Autodesk Inventor part; units mm, degrees
(part 2 of 4)
  spline S285 degree 2 poles (64.2281, 27.9943) (64.3898, 27.9943) (64.7103, 28.0368) (64.8067, 28.0822) knots 0 0 0 1 2 2 2
  spline S286 degree 2 poles (64.8067, 28.0822) (64.9173, 28.1389) (65.0421, 28.329) (65.0534, 28.4708) knots 0 0 0 1 2 2 2
  line L243 (65.0534, 28.4708) -> (65.8192, 28.4708)
  line L244 (65.8192, 28.4708) -> (65.8192, 25.5721)
  line L245 (65.8192, 25.5721) -> (66.5397, 25.5721)
  line L246 (66.5397, 25.5721) -> (66.5397, 24.9623)
  line L247 (69.1803, 28.6183) -> (67.7876, 24.2021)
  line L248 (67.7876, 24.2021) -> (67.1126, 24.2021)
  line L249 (67.1126, 24.2021) -> (68.5024, 28.6183)
  line L250 (68.5024, 28.6183) -> (69.1803, 28.6183)
  spline S287 degree 2 poles (71.4833, 24.8942) (70.6949, 24.8942) (69.7702, 25.8472) (69.7702, 26.7094) knots 0 0 0 1 2 2 2
  spline S288 degree 2 poles (69.7702, 26.7094) (69.7702, 27.5405) (70.6977, 28.5303) (71.4862, 28.5303) knots 0 0 0 1 2 2 2
  spline S289 degree 2 poles (71.4862, 28.5303) (71.6932, 28.5303) (72.0279, 28.4821) (72.1811, 28.4424) knots 0 0 0 1 2 2 2
  spline S290 degree 2 poles (72.1811, 28.4424) (72.3002, 28.4055) (72.581, 28.2836) (72.6689, 28.2382) knots 0 0 0 1 2 2 2
  line L251 (72.6689, 28.2382) -> (72.6689, 27.4043)
  line L252 (72.6689, 27.4043) -> (72.581, 27.4043)
  spline S291 degree 2 poles (72.581, 27.4043) (72.5158, 27.461) (72.3229, 27.6199) (72.2009, 27.6936) knots 0 0 0 1 2 2 2
  spline S292 degree 2 poles (72.2009, 27.6936) (72.079, 27.7702) (71.7868, 27.8751) (71.6252, 27.8751) knots 0 0 0 1 2 2 2
  spline S293 degree 2 poles (71.6252, 27.8751) (71.4351, 27.8751) (71.1203, 27.756) (70.9757, 27.6057) knots 0 0 0 1 2 2 2
  spline S294 degree 2 poles (70.9757, 27.6057) (70.8452, 27.4724) (70.6778, 27.0157) (70.6778, 26.7066) knots 0 0 0 1 2 2 2
  spline S295 degree 2 poles (70.6778, 26.7066) (70.6778, 26.3804) (70.8509, 25.9351) (70.9927, 25.799) knots 0 0 0 1 2 2 2
  spline S296 degree 2 poles (70.9927, 25.799) (71.1288, 25.6657) (71.4635, 25.5494) (71.6308, 25.5494) knots 0 0 0 1 2 2 2
  spline S297 degree 2 poles (71.6308, 25.5494) (71.8039, 25.5494) (72.1187, 25.6657) (72.2265, 25.7366) knots 0 0 0 1 2 2 2
  spline S298 degree 2 poles (72.2265, 25.7366) (72.3456, 25.8075) (72.5243, 25.9578) (72.5895, 26.0174) knots 0 0 0 1 2 2 2
  line L253 (72.5895, 26.0174) -> (72.6689, 26.0174)
  line L254 (72.6689, 26.0174) -> (72.6689, 25.1948)
  spline S299 degree 2 poles (72.6689, 25.1948) (72.5725, 25.1495) (72.3201, 25.036) (72.1839, 24.9963) knots 0 0 0 1 2 2 2
  spline S300 degree 2 poles (72.1839, 24.9963) (72.0194, 24.9452) (71.7329, 24.8942) (71.4833, 24.8942) knots 0 0 0 1 2 2 2
  spline S301 degree 2 poles (74.5948, 25.2431) (74.5097, 25.1721) (74.3764, 25.0587) (74.2629, 25.002) knots 0 0 0 1 2 2 2
  spline S302 degree 2 poles (74.2629, 25.002) (74.1523, 24.9481) (73.9424, 24.8914) (73.7552, 24.8914) knots 0 0 0 1 2 2 2
  spline S303 degree 2 poles (73.7552, 24.8914) (73.4035, 24.8914) (72.9412, 25.3622) (72.9412, 25.7196) knots 0 0 0 1 2 2 2
  spline S304 degree 2 poles (72.9412, 25.7196) (72.9412, 26.0117) (73.1766, 26.3747) (73.3979, 26.4797) knots 0 0 0 1 2 2 2
  spline S305 degree 2 poles (73.3979, 26.4797) (73.6219, 26.5875) (74.2431, 26.6726) (74.6004, 26.6952) knots 0 0 0 1 2 2 2
  line L255 (74.6004, 26.6952) -> (74.6004, 26.7094)
  spline S306 degree 2 poles (74.6004, 26.7094) (74.6004, 26.9278) (74.2771, 27.0952) (73.9538, 27.0952) knots 0 0 0 1 2 2 2
  spline S307 degree 2 poles (73.9538, 27.0952) (73.8091, 27.0952) (73.4177, 26.9902) (73.2333, 26.908) knots 0 0 0 1 2 2 2
  line L256 (73.2333, 26.908) -> (73.1624, 26.908)
  line L257 (73.1624, 26.908) -> (73.1624, 27.5461)
  spline S308 degree 2 poles (73.1624, 27.5461) (73.2844, 27.5802) (73.829, 27.6766) (74.1069, 27.6766) knots 0 0 0 1 2 2 2
  spline S309 degree 2 poles (74.1069, 27.6766) (74.7876, 27.6766) (75.4116, 27.2228) (75.4116, 26.7576) knots 0 0 0 1 2 2 2
  line L258 (75.4116, 26.7576) -> (75.4116, 24.9623)
  line L259 (75.4116, 24.9623) -> (74.5948, 24.9623)
  line L260 (74.5948, 24.9623) -> (74.5948, 25.2431)
  line L261 (74.5948, 25.6515) -> (74.5948, 26.1989)
  spline S310 degree 2 poles (74.5948, 26.1989) (74.3849, 26.179) (74.1268, 26.1478) (74.002, 26.1025) knots 0 0 0 1 2 2 2
  spline S311 degree 2 poles (74.002, 26.1025) (73.8914, 26.0656) (73.7722, 25.9124) (73.7722, 25.7876) knots 0 0 0 1 2 2 2
  spline S312 degree 2 poles (73.7722, 25.7876) (73.7722, 25.6033) (73.9736, 25.4643) (74.1693, 25.4643) knots 0 0 0 1 2 2 2
  spline S313 degree 2 poles (74.1693, 25.4643) (74.2771, 25.4643) (74.504, 25.5636) (74.5948, 25.6515) knots 0 0 0 1 2 2 2
  line L262 (76.844, 24.9623) -> (76.0214, 24.9623)
  line L263 (76.0214, 24.9623) -> (76.0214, 28.6183)
  line L264 (76.0214, 28.6183) -> (76.844, 28.6183)
  line L265 (76.844, 28.6183) -> (76.844, 24.9623)
  spline S314 degree 2 poles (80.0064, 26.2811) (80.0064, 25.6288) (79.2945, 24.88) (78.645, 24.88) knots 0 0 0 1 2 2 2
  spline S315 degree 2 poles (78.645, 24.88) (77.9983, 24.88) (77.2808, 25.6288) (77.2808, 26.2811) knots 0 0 0 1 2 2 2
  spline S316 degree 2 poles (77.2808, 26.2811) (77.2808, 26.9392) (77.9983, 27.6851) (78.645, 27.6851) knots 0 0 0 1 2 2 2
  spline S317 degree 2 poles (78.645, 27.6851) (79.2917, 27.6851) (80.0064, 26.9363) (80.0064, 26.2811) knots 0 0 0 1 2 2 2
  spline S318 degree 2 poles (79.1641, 26.2755) (79.1641, 26.5109) (79.0875, 26.8257) (79.0194, 26.9193) knots 0 0 0 1 2 2 2
  spline S319 degree 2 poles (79.0194, 26.9193) (78.9457, 27.0186) (78.7613, 27.0952) (78.645, 27.0952) knots 0 0 0 1 2 2 2
  spline S320 degree 2 poles (78.645, 27.0952) (78.5316, 27.0952) (78.3529, 27.0271) (78.2791, 26.9307) knots 0 0 0 1 2 2 2
  spline S321 degree 2 poles (78.2791, 26.9307) (78.2082, 26.8399) (78.1231, 26.5194) (78.1231, 26.2755) knots 0 0 0 1 2 2 2
  spline S322 degree 2 poles (78.1231, 26.2755) (78.1231, 26.0344) (78.2026, 25.7366) (78.2678, 25.6458) knots 0 0 0 1 2 2 2
  spline S323 degree 2 poles (78.2678, 25.6458) (78.333, 25.555) (78.5316, 25.47) (78.6507, 25.47) knots 0 0 0 1 2 2 2
  spline S324 degree 2 poles (78.6507, 25.47) (78.75, 25.47) (78.9542, 25.555) (79.0166, 25.6401) knots 0 0 0 1 2 2 2
  spline S325 degree 2 poles (79.0166, 25.6401) (79.0875, 25.7394) (79.1641, 26.0259) (79.1641, 26.2755) knots 0 0 0 1 2 2 2
  line L266 (82.2159, 26.8229) -> (82.1479, 26.8229)
  spline S326 degree 2 poles (82.1479, 26.8229) (82.0996, 26.8399) (81.921, 26.8569) (81.8132, 26.8569) knots 0 0 0 1 2 2 2
  spline S327 degree 2 poles (81.8132, 26.8569) (81.6855, 26.8569) (81.3991, 26.7803) (81.2658, 26.7293) knots 0 0 0 1 2 2 2
  line L267 (81.2658, 26.7293) -> (81.2658, 24.9623)
  line L268 (81.2658, 24.9623) -> (80.4432, 24.9623)
  line L269 (80.4432, 24.9623) -> (80.4432, 27.6029)
  line L270 (80.4432, 27.6029) -> (81.2658, 27.6029)
  line L271 (81.2658, 27.6029) -> (81.2658, 27.2228)
  spline S328 degree 2 poles (81.2658, 27.2228) (81.3225, 27.2739) (81.521, 27.4327) (81.6033, 27.4809) knots 0 0 0 1 2 2 2
  spline S329 degree 2 poles (81.6033, 27.4809) (81.694, 27.5348) (81.9323, 27.6114) (82.0372, 27.6114) knots 0 0 0 1 2 2 2
  spline S330 degree 2 poles (82.0372, 27.6114) (82.0769, 27.6114) (82.1762, 27.6057) (82.2159, 27.6029) knots 0 0 0 1 2 2 2
  line L272 (82.2159, 27.6029) -> (82.2159, 26.8229)
  line L273 (83.3533, 24.9623) -> (82.5308, 24.9623)
  line L274 (82.5308, 24.9623) -> (82.5308, 27.6029)
  line L275 (82.5308, 27.6029) -> (83.3533, 27.6029)
  line L276 (83.3533, 27.6029) -> (83.3533, 24.9623)
  line L277 (83.3788, 27.9801) -> (82.5081, 27.9801)
  line L278 (82.5081, 27.9801) -> (82.5081, 28.6211)
  line L279 (82.5081, 28.6211) -> (83.3788, 28.6211)
  line L280 (83.3788, 28.6211) -> (83.3788, 27.9801)
  line L281 (87.1341, 24.9623) -> (87.1341, 26.2811)
  spline S331 degree 2 poles (87.1341, 26.2811) (87.1341, 26.4768) (87.1199, 26.7435) (87.0859, 26.8286) knots 0 0 0 1 2 2 2
  spline S332 degree 2 poles (87.0859, 26.8286) (87.049, 26.9136) (86.9015, 26.9902) (86.7682, 26.9902) knots 0 0 0 1 2 2 2
  spline S333 degree 2 poles (86.7682, 26.9902) (86.6746, 26.9902) (86.4931, 26.908) (86.3853, 26.8314) knots 0 0 0 1 2 2 2
  line L282 (86.3853, 26.8314) -> (86.3853, 24.9623)
  line L283 (86.3853, 24.9623) -> (85.5571, 24.9623)
  line L284 (85.5571, 24.9623) -> (85.5571, 26.2811)
  spline S334 degree 2 poles (85.5571, 26.2811) (85.5571, 26.474) (85.5401, 26.7435) (85.506, 26.8286) knots 0 0 0 1 2 2 2
  spline S335 degree 2 poles (85.506, 26.8286) (85.4692, 26.9136) (85.3217, 26.9902) (85.1884, 26.9902) knots 0 0 0 1 2 2 2
  spline S336 degree 2 poles (85.1884, 26.9902) (85.0891, 26.9902) (84.8934, 26.8966) (84.8026, 26.8314) knots 0 0 0 1 2 2 2
  line L285 (84.8026, 26.8314) -> (84.8026, 24.9623)
  line L286 (84.8026, 24.9623) -> (83.9801, 24.9623)
  line L287 (83.9801, 24.9623) -> (83.9801, 27.6029)
  line L288 (83.9801, 27.6029) -> (84.8026, 27.6029)
  line L289 (84.8026, 27.6029) -> (84.8026, 27.3107)
  spline S337 degree 2 poles (84.8026, 27.3107) (85.004, 27.4809) (85.3642, 27.6738) (85.5883, 27.6738) knots 0 0 0 1 2 2 2
  spline S338 degree 2 poles (85.5883, 27.6738) (85.8294, 27.6738) (86.1981, 27.444) (86.2945, 27.2143) knots 0 0 0 1 2 2 2
  spline S339 degree 2 poles (86.2945, 27.2143) (86.5299, 27.4355) (86.9497, 27.6738) (87.1653, 27.6738) knots 0 0 0 1 2 2 2
  spline S340 degree 2 poles (87.1653, 27.6738) (87.3496, 27.6738) (87.6418, 27.5575) (87.741, 27.4384) knots 0 0 0 1 2 2 2
  spline S341 degree 2 poles (87.741, 27.4384) (87.8517, 27.3107) (87.9623, 26.9619) (87.9623, 26.6811) knots 0 0 0 1 2 2 2
  line L290 (87.9623, 26.6811) -> (87.9623, 24.9623)
  line L291 (87.9623, 24.9623) -> (87.1341, 24.9623)
  spline S342 degree 2 poles (89.925, 24.8914) (89.1762, 24.8914) (88.3792, 25.6061) (88.3792, 26.267) knots 0 0 0 1 2 2 2
  spline S343 degree 2 poles (88.3792, 26.267) (88.3792, 26.9136) (89.1223, 27.6851) (89.7917, 27.6851) knots 0 0 0 1 2 2 2
  spline S344 degree 2 poles (89.7917, 27.6851) (90.3958, 27.6851) (91.0085, 27.0299) (91.0085, 26.423) knots 0 0 0 1 2 2 2
  line L292 (91.0085, 26.423) -> (91.0085, 26.1251)
  line L293 (91.0085, 26.1251) -> (89.2017, 26.1251)
  spline S345 degree 2 poles (89.2017, 26.1251) (89.2131, 25.9408) (89.3464, 25.6969) (89.4542, 25.6231) knots 0 0 0 1 2 2 2
  spline S346 degree 2 poles (89.4542, 25.6231) (89.5591, 25.5494) (89.8427, 25.487) (90.0101, 25.487) knots 0 0 0 1 2 2 2
  spline S347 degree 2 poles (90.0101, 25.487) (90.1519, 25.487) (90.4299, 25.5494) (90.5462, 25.6033) knots 0 0 0 1 2 2 2
  spline S348 degree 2 poles (90.5462, 25.6033) (90.6483, 25.6458) (90.8184, 25.7508) (90.8723, 25.7905) knots 0 0 0 1 2 2 2
  line L294 (90.8723, 25.7905) -> (90.9603, 25.7905)
  line L295 (90.9603, 25.7905) -> (90.9603, 25.1097)
  spline S349 degree 2 poles (90.9603, 25.1097) (90.8581, 25.07) (90.6936, 25.002) (90.5462, 24.9679) knots 0 0 0 1 2 2 2
  spline S350 degree 2 poles (90.5462, 24.9679) (90.4128, 24.9311) (90.1292, 24.8914) (89.925, 24.8914) knots 0 0 0 1 2 2 2
  spline S351 degree 2 poles (90.1973, 26.6215) (90.1916, 26.8824) (89.9619, 27.1576) (89.7265, 27.1576) knots 0 0 0 1 2 2 2
  spline S352 degree 2 poles (89.7265, 27.1576) (89.4854, 27.1576) (89.2131, 26.8683) (89.1989, 26.6215) knots 0 0 0 1 2 2 2
  line L296 (89.1989, 26.6215) -> (90.1973, 26.6215)
  spline S353 degree 2 poles (92.4408, 24.9112) (91.9388, 24.9112) (91.4793, 25.3253) (91.4793, 25.7961) knots 0 0 0 1 2 2 2
  line L297 (91.4793, 25.7961) -> (91.4793, 27.0299)
  line L298 (91.4793, 27.0299) -> (91.1645, 27.0299)
  line L299 (91.1645, 27.0299) -> (91.1645, 27.6029)
  line L300 (91.1645, 27.6029) -> (91.4793, 27.6029)
  line L301 (91.4793, 27.6029) -> (91.4793, 28.3573)
  line L302 (91.4793, 28.3573) -> (92.3018, 28.3573)
  line L303 (92.3018, 28.3573) -> (92.3018, 27.6029)
  line L304 (92.3018, 27.6029) -> (93.096, 27.6029)
  line L305 (93.096, 27.6029) -> (93.096, 27.0299)
  line L306 (93.096, 27.0299) -> (92.3018, 27.0299)
  line L307 (92.3018, 27.0299) -> (92.3018, 26.0911)
  spline S354 degree 2 poles (92.3018, 26.0911) (92.3018, 25.9521) (92.3075, 25.7451) (92.3415, 25.6628) knots 0 0 0 1 2 2 2
  spline S355 degree 2 poles (92.3415, 25.6628) (92.3756, 25.5806) (92.5429, 25.4841) (92.7017, 25.4841) knots 0 0 0 1 2 2 2
  spline S356 degree 2 poles (92.7017, 25.4841) (92.7698, 25.4841) (92.9825, 25.5409) (93.0251, 25.5636) knots 0 0 0 1 2 2 2
  line L308 (93.0251, 25.5636) -> (93.096, 25.5636)
  line L309 (93.096, 25.5636) -> (93.096, 24.985)
  spline S357 degree 2 poles (93.096, 24.985) (92.9627, 24.9509) (92.662, 24.9112) (92.4408, 24.9112) knots 0 0 0 1 2 2 2
  line L310 (95.2034, 26.8229) -> (95.1353, 26.8229)
  spline S358 degree 2 poles (95.1353, 26.8229) (95.0871, 26.8399) (94.9084, 26.8569) (94.8006, 26.8569) knots 0 0 0 1 2 2 2
  spline S359 degree 2 poles (94.8006, 26.8569) (94.673, 26.8569) (94.3865, 26.7803) (94.2532, 26.7293) knots 0 0 0 1 2 2 2
  line L311 (94.2532, 26.7293) -> (94.2532, 24.9623)
  line L312 (94.2532, 24.9623) -> (93.4307, 24.9623)
  line L313 (93.4307, 24.9623) -> (93.4307, 27.6029)
  line L314 (93.4307, 27.6029) -> (94.2532, 27.6029)
  line L315 (94.2532, 27.6029) -> (94.2532, 27.2228)
  spline S360 degree 2 poles (94.2532, 27.2228) (94.3099, 27.2739) (94.5085, 27.4327) (94.5907, 27.4809) knots 0 0 0 1 2 2 2
  spline S361 degree 2 poles (94.5907, 27.4809) (94.6815, 27.5348) (94.9197, 27.6114) (95.0247, 27.6114) knots 0 0 0 1 2 2 2
  spline S362 degree 2 poles (95.0247, 27.6114) (95.0644, 27.6114) (95.1637, 27.6057) (95.2034, 27.6029) knots 0 0 0 1 2 2 2
  line L316 (95.2034, 27.6029) -> (95.2034, 26.8229)
  spline S363 degree 2 poles (98.051, 26.2811) (98.051, 25.6288) (97.3391, 24.88) (96.6896, 24.88) knots 0 0 0 1 2 2 2
  spline S364 degree 2 poles (96.6896, 24.88) (96.0429, 24.88) (95.3253, 25.6288) (95.3253, 26.2811) knots 0 0 0 1 2 2 2
  spline S365 degree 2 poles (95.3253, 26.2811) (95.3253, 26.9392) (96.0429, 27.6851) (96.6896, 27.6851) knots 0 0 0 1 2 2 2
  spline S366 degree 2 poles (96.6896, 27.6851) (97.3363, 27.6851) (98.051, 26.9363) (98.051, 26.2811) knots 0 0 0 1 2 2 2
  spline S367 degree 2 poles (97.2086, 26.2755) (97.2086, 26.5109) (97.1321, 26.8257) (97.064, 26.9193) knots 0 0 0 1 2 2 2
  spline S368 degree 2 poles (97.064, 26.9193) (96.9902, 27.0186) (96.8059, 27.0952) (96.6896, 27.0952) knots 0 0 0 1 2 2 2
  spline S369 degree 2 poles (96.6896, 27.0952) (96.5761, 27.0952) (96.3974, 27.0271) (96.3237, 26.9307) knots 0 0 0 1 2 2 2
  spline S370 degree 2 poles (96.3237, 26.9307) (96.2528, 26.8399) (96.1677, 26.5194) (96.1677, 26.2755) knots 0 0 0 1 2 2 2
  spline S371 degree 2 poles (96.1677, 26.2755) (96.1677, 26.0344) (96.2471, 25.7366) (96.3124, 25.6458) knots 0 0 0 1 2 2 2
  spline S372 degree 2 poles (96.3124, 25.6458) (96.3776, 25.555) (96.5761, 25.47) (96.6953, 25.47) knots 0 0 0 1 2 2 2
  spline S373 degree 2 poles (96.6953, 25.47) (96.7945, 25.47) (96.9987, 25.555) (97.0611, 25.6401) knots 0 0 0 1 2 2 2
  spline S374 degree 2 poles (97.0611, 25.6401) (97.1321, 25.7394) (97.2086, 26.0259) (97.2086, 26.2755) knots 0 0 0 1 2 2 2
  spline S375 degree 2 poles (27.7919, 16.1032) (27.5359, 15.9989) (26.7174, 15.7998) (26.3191, 15.7998) knots 0 0 0 1 2 2 2
  spline S376 degree 2 poles (26.3191, 15.7998) (25.3994, 15.7998) (24.3091, 16.8617) (24.3091, 17.8351) knots 0 0 0 1 2 2 2
  spline S377 degree 2 poles (24.3091, 17.8351) (24.3091, 18.7517) (25.3994, 19.8578) (26.3476, 19.8578) knots 0 0 0 1 2 2 2
  spline S378 degree 2 poles (26.3476, 19.8578) (26.8374, 19.8578) (27.4506, 19.6714) (27.7761, 19.5133) knots 0 0 0 1 2 2 2
  line L317 (27.7761, 19.5133) -> (27.7761, 18.5968)
  line L318 (27.7761, 18.5968) -> (27.6876, 18.5968)
  spline S379 degree 2 poles (27.6876, 18.5968) (27.6181, 18.6505) (27.3526, 18.856) (27.2262, 18.9255) knots 0 0 0 1 2 2 2
  spline S380 degree 2 poles (27.2262, 18.9255) (27.0808, 19.0108) (26.6952, 19.1309) (26.4803, 19.1309) knots 0 0 0 1 2 2 2
  spline S381 degree 2 poles (26.4803, 19.1309) (26.2306, 19.1309) (25.8166, 18.9729) (25.6554, 18.8117) knots 0 0 0 1 2 2 2
  spline S382 degree 2 poles (25.6554, 18.8117) (25.5006, 18.6537) (25.3204, 18.1701) (25.3204, 17.8509) knots 0 0 0 1 2 2 2
  spline S383 degree 2 poles (25.3204, 17.8509) (25.3204, 17.1683) (26.0062, 16.5172) (26.5973, 16.5172) knots 0 0 0 1 2 2 2
  spline S384 degree 2 poles (26.5973, 16.5172) (26.651, 16.5172) (26.79, 16.5235) (26.8438, 16.5267) knots 0 0 0 1 2 2 2
  line L319 (26.8438, 16.5267) -> (26.8438, 17.2947)
  line L320 (26.8438, 17.2947) -> (26.0884, 17.2947)
  line L321 (26.0884, 17.2947) -> (26.0884, 18.0248)
  line L322 (26.0884, 18.0248) -> (27.7919, 18.0248)
  line L323 (27.7919, 18.0248) -> (27.7919, 16.1032)
  spline S385 degree 2 poles (30.099, 16.1949) (30.0042, 16.1158) (29.8557, 15.9894) (29.7293, 15.9262) knots 0 0 0 1 2 2 2
  spline S386 degree 2 poles (29.7293, 15.9262) (29.606, 15.8662) (29.3721, 15.803) (29.1635, 15.803) knots 0 0 0 1 2 2 2
  spline S387 degree 2 poles (29.1635, 15.803) (28.7716, 15.803) (28.2565, 16.3276) (28.2565, 16.7258) knots 0 0 0 1 2 2 2
  spline S388 degree 2 poles (28.2565, 16.7258) (28.2565, 17.0513) (28.5188, 17.4559) (28.7653, 17.5728) knots 0 0 0 1 2 2 2
  spline S389 degree 2 poles (28.7653, 17.5728) (29.015, 17.6929) (29.7071, 17.7877) (30.1054, 17.813) knots 0 0 0 1 2 2 2
  line L324 (30.1054, 17.813) -> (30.1054, 17.8288)
  spline S390 degree 2 poles (30.1054, 17.8288) (30.1054, 18.0722) (29.7451, 18.2586) (29.3848, 18.2586) knots 0 0 0 1 2 2 2
  spline S391 degree 2 poles (29.3848, 18.2586) (29.2236, 18.2586) (28.7874, 18.1417) (28.582, 18.05) knots 0 0 0 1 2 2 2
  line L325 (28.582, 18.05) -> (28.503, 18.05)
  line L326 (28.503, 18.05) -> (28.503, 18.7611)
  spline S392 degree 2 poles (28.503, 18.7611) (28.6389, 18.7991) (29.2457, 18.9065) (29.5554, 18.9065) knots 0 0 0 1 2 2 2
  spline S393 degree 2 poles (29.5554, 18.9065) (30.3139, 18.9065) (31.0092, 18.4009) (31.0092, 17.8825) knots 0 0 0 1 2 2 2
  line L327 (31.0092, 17.8825) -> (31.0092, 15.882)
  line L328 (31.0092, 15.882) -> (30.099, 15.882)
  line L329 (30.099, 15.882) -> (30.099, 16.1949)
  line L330 (30.099, 16.65) -> (30.099, 17.2599)
  spline S394 degree 2 poles (30.099, 17.2599) (29.8652, 17.2378) (29.5776, 17.203) (29.4385, 17.1525) knots 0 0 0 1 2 2 2
  spline S395 degree 2 poles (29.4385, 17.1525) (29.3152, 17.1114) (29.1825, 16.9407) (29.1825, 16.8017) knots 0 0 0 1 2 2 2
  spline S396 degree 2 poles (29.1825, 16.8017) (29.1825, 16.5962) (29.4069, 16.4414) (29.625, 16.4414) knots 0 0 0 1 2 2 2
  spline S397 degree 2 poles (29.625, 16.4414) (29.7451, 16.4414) (29.9979, 16.552) (30.099, 16.65) knots 0 0 0 1 2 2 2
  spline S398 degree 2 poles (34.5711, 17.3927) (34.5711, 16.6911) (33.86, 15.8251) (33.3322, 15.8251) knots 0 0 0 1 2 2 2
  spline S399 degree 2 poles (33.3322, 15.8251) (33.1141, 15.8251) (32.7886, 15.9231) (32.6053, 16.0274) knots 0 0 0 1 2 2 2
  line L331 (32.6053, 16.0274) -> (32.5674, 15.882)
  line L332 (32.5674, 15.882) -> (31.6887, 15.882)
  line L333 (31.6887, 15.882) -> (31.6887, 19.9558)
  line L334 (31.6887, 19.9558) -> (32.6053, 19.9558)
  line L335 (32.6053, 19.9558) -> (32.6053, 18.5146)
  spline S400 degree 2 poles (32.6053, 18.5146) (32.8075, 18.6885) (33.2247, 18.9034) (33.4997, 18.9034) knots 0 0 0 1 2 2 2
  spline S401 degree 2 poles (33.4997, 18.9034) (34.0148, 18.9034) (34.5711, 18.1038) (34.5711, 17.3927) knots 0 0 0 1 2 2 2
  spline S402 degree 2 poles (33.6324, 17.3737) (33.6324, 17.813) (33.3669, 18.1891) (33.0888, 18.1891) knots 0 0 0 1 2 2 2
  spline S403 degree 2 poles (33.0888, 18.1891) (32.9656, 18.1891) (32.7222, 18.1101) (32.6053, 18.0311) knots 0 0 0 1 2 2 2
  line L336 (32.6053, 18.0311) -> (32.6053, 16.5583)
  spline S404 degree 2 poles (32.6053, 16.5583) (32.6969, 16.5204) (32.8834, 16.4951) (32.975, 16.4951) knots 0 0 0 1 2 2 2
  spline S405 degree 2 poles (32.975, 16.4951) (33.3069, 16.4951) (33.6324, 16.9344) (33.6324, 17.3737) knots 0 0 0 1 2 2 2
  line L337 (37.052, 17.9552) -> (36.9762, 17.9552)
  spline S406 degree 2 poles (36.9762, 17.9552) (36.9225, 17.9742) (36.7233, 17.9932) (36.6033, 17.9932) knots 0 0 0 1 2 2 2
  spline S407 degree 2 poles (36.6033, 17.9932) (36.461, 17.9932) (36.1418, 17.9078) (35.9933, 17.8509) knots 0 0 0 1 2 2 2
  line L338 (35.9933, 17.8509) -> (35.9933, 15.882)
  line L339 (35.9933, 15.882) -> (35.0768, 15.882)
  line L340 (35.0768, 15.882) -> (35.0768, 18.8244)
  line L341 (35.0768, 18.8244) -> (35.9933, 18.8244)
  line L342 (35.9933, 18.8244) -> (35.9933, 18.4009)
  spline S408 degree 2 poles (35.9933, 18.4009) (36.0565, 18.4577) (36.2777, 18.6347) (36.3694, 18.6885) knots 0 0 0 1 2 2 2
  spline S409 degree 2 poles (36.3694, 18.6885) (36.4705, 18.7485) (36.736, 18.8338) (36.8529, 18.8338) knots 0 0 0 1 2 2 2
  spline S410 degree 2 poles (36.8529, 18.8338) (36.8972, 18.8338) (37.0078, 18.8275) (37.052, 18.8244) knots 0 0 0 1 2 2 2
  line L343 (37.052, 18.8244) -> (37.052, 17.9552)
  line L344 (38.3194, 15.882) -> (37.4028, 15.882)
  line L345 (37.4028, 15.882) -> (37.4028, 18.8244)
  line L346 (37.4028, 18.8244) -> (38.3194, 18.8244)
  line L347 (38.3194, 18.8244) -> (38.3194, 15.882)
  line L348 (38.3478, 19.2447) -> (37.3776, 19.2447)
  line L349 (37.3776, 19.2447) -> (37.3776, 19.959)
  line L350 (37.3776, 19.959) -> (38.3478, 19.959)
  line L351 (38.3478, 19.959) -> (38.3478, 19.2447)
  spline S411 degree 2 poles (40.5285, 15.803) (39.6942, 15.803) (38.8061, 16.5994) (38.8061, 17.3358) knots 0 0 0 1 2 2 2
  spline S412 degree 2 poles (38.8061, 17.3358) (38.8061, 18.0564) (39.6341, 18.916) (40.38, 18.916) knots 0 0 0 1 2 2 2
  spline S413 degree 2 poles (40.38, 18.916) (41.0532, 18.916) (41.7358, 18.1859) (41.7358, 17.5096) knots 0 0 0 1 2 2 2
  line L352 (41.7358, 17.5096) -> (41.7358, 17.1778)
  line L353 (41.7358, 17.1778) -> (39.7226, 17.1778)
  spline S414 degree 2 poles (39.7226, 17.1778) (39.7353, 16.9723) (39.8838, 16.7005) (40.0039, 16.6184) knots 0 0 0 1 2 2 2
  spline S415 degree 2 poles (40.0039, 16.6184) (40.1208, 16.5362) (40.4369, 16.4667) (40.6233, 16.4667) knots 0 0 0 1 2 2 2
  spline S416 degree 2 poles (40.6233, 16.4667) (40.7814, 16.4667) (41.0911, 16.5362) (41.2207, 16.5962) knots 0 0 0 1 2 2 2
  spline S417 degree 2 poles (41.2207, 16.5962) (41.3344, 16.6436) (41.5241, 16.7606) (41.5841, 16.8048) knots 0 0 0 1 2 2 2
  line L354 (41.5841, 16.8048) -> (41.6821, 16.8048)
  line L355 (41.6821, 16.8048) -> (41.6821, 16.0463)
  spline S418 degree 2 poles (41.6821, 16.0463) (41.5683, 16.0021) (41.385, 15.9262) (41.2207, 15.8883) knots 0 0 0 1 2 2 2
  spline S419 degree 2 poles (41.2207, 15.8883) (41.0721, 15.8472) (40.7561, 15.803) (40.5285, 15.803) knots 0 0 0 1 2 2 2
  spline S420 degree 2 poles (40.8319, 17.7308) (40.8256, 18.0216) (40.5696, 18.3282) (40.3073, 18.3282) knots 0 0 0 1 2 2 2
  spline S421 degree 2 poles (40.3073, 18.3282) (40.0387, 18.3282) (39.7353, 18.0058) (39.7195, 17.7308) knots 0 0 0 1 2 2 2
  line L356 (39.7195, 17.7308) -> (40.8319, 17.7308)
  line L357 (43.1233, 15.882) -> (42.2067, 15.882)
  line L358 (42.2067, 15.882) -> (42.2067, 19.9558)
  line L359 (42.2067, 19.9558) -> (43.1233, 19.9558)
  line L360 (43.1233, 19.9558) -> (43.1233, 15.882)
  spline S422 degree 2 poles (47.1307, 15.8061) (46.2521, 15.8061) (45.2218, 16.868) (45.2218, 17.8288) knots 0 0 0 1 2 2 2
  spline S423 degree 2 poles (45.2218, 17.8288) (45.2218, 18.7548) (46.2553, 19.8578) (47.1339, 19.8578) knots 0 0 0 1 2 2 2
  spline S424 degree 2 poles (47.1339, 19.8578) (47.3646, 19.8578) (47.7375, 19.8041) (47.9082, 19.7599) knots 0 0 0 1 2 2 2
  spline S425 degree 2 poles (47.9082, 19.7599) (48.0409, 19.7188) (48.3538, 19.5829) (48.4518, 19.5323) knots 0 0 0 1 2 2 2
  line L361 (48.4518, 19.5323) -> (48.4518, 18.6031)
  line L362 (48.4518, 18.6031) -> (48.3538, 18.6031)
  spline S426 degree 2 poles (48.3538, 18.6031) (48.2811, 18.6663) (48.0662, 18.8433) (47.9303, 18.9255) knots 0 0 0 1 2 2 2
  spline S427 degree 2 poles (47.9303, 18.9255) (47.7944, 19.0108) (47.4689, 19.1278) (47.2887, 19.1278) knots 0 0 0 1 2 2 2
  spline S428 degree 2 poles (47.2887, 19.1278) (47.077, 19.1278) (46.7262, 18.995) (46.565, 18.8275) knots 0 0 0 1 2 2 2
  spline S429 degree 2 poles (46.565, 18.8275) (46.4196, 18.679) (46.2332, 18.1701) (46.2332, 17.8257) knots 0 0 0 1 2 2 2
  spline S430 degree 2 poles (46.2332, 17.8257) (46.2332, 17.4622) (46.4259, 16.966) (46.584, 16.8143) knots 0 0 0 1 2 2 2
  spline S431 degree 2 poles (46.584, 16.8143) (46.7357, 16.6658) (47.1086, 16.5362) (47.2951, 16.5362) knots 0 0 0 1 2 2 2
  spline S432 degree 2 poles (47.2951, 16.5362) (47.4879, 16.5362) (47.8387, 16.6658) (47.9588, 16.7448) knots 0 0 0 1 2 2 2
  spline S433 degree 2 poles (47.9588, 16.7448) (48.0915, 16.8238) (48.2906, 16.9913) (48.3633, 17.0577) knots 0 0 0 1 2 2 2
  line L363 (48.3633, 17.0577) -> (48.4518, 17.0577)
  line L364 (48.4518, 17.0577) -> (48.4518, 16.1411)
  spline S434 degree 2 poles (48.4518, 16.1411) (48.3443, 16.0906) (48.0631, 15.9641) (47.9114, 15.9199) knots 0 0 0 1 2 2 2
  spline S435 degree 2 poles (47.9114, 15.9199) (47.728, 15.863) (47.4088, 15.8061) (47.1307, 15.8061) knots 0 0 0 1 2 2 2
  spline S436 degree 2 poles (51.7987, 17.3516) (51.7987, 16.6247) (51.0054, 15.7903) (50.2817, 15.7903) knots 0 0 0 1 2 2 2
  spline S437 degree 2 poles (50.2817, 15.7903) (49.5611, 15.7903) (48.7615, 16.6247) (48.7615, 17.3516) knots 0 0 0 1 2 2 2
  spline S438 degree 2 poles (48.7615, 17.3516) (48.7615, 18.0848) (49.5611, 18.916) (50.2817, 18.916) knots 0 0 0 1 2 2 2
  spline S439 degree 2 poles (50.2817, 18.916) (51.0023, 18.916) (51.7987, 18.0817) (51.7987, 17.3516) knots 0 0 0 1 2 2 2
  spline S440 degree 2 poles (50.8601, 17.3453) (50.8601, 17.6076) (50.7747, 17.9584) (50.6989, 18.0627) knots 0 0 0 1 2 2 2
  spline S441 degree 2 poles (50.6989, 18.0627) (50.6167, 18.1733) (50.4113, 18.2586) (50.2817, 18.2586) knots 0 0 0 1 2 2 2
  spline S442 degree 2 poles (50.2817, 18.2586) (50.1553, 18.2586) (49.9562, 18.1828) (49.874, 18.0753) knots 0 0 0 1 2 2 2
  spline S443 degree 2 poles (49.874, 18.0753) (49.795, 17.9742) (49.7002, 17.6171) (49.7002, 17.3453) knots 0 0 0 1 2 2 2
  spline S444 degree 2 poles (49.7002, 17.3453) (49.7002, 17.0766) (49.7887, 16.7448) (49.8614, 16.6436) knots 0 0 0 1 2 2 2
  spline S445 degree 2 poles (49.8614, 16.6436) (49.934, 16.5425) (50.1553, 16.4477) (50.288, 16.4477) knots 0 0 0 1 2 2 2
  spline S446 degree 2 poles (50.288, 16.4477) (50.3986, 16.4477) (50.6262, 16.5425) (50.6957, 16.6373) knots 0 0 0 1 2 2 2
  spline S447 degree 2 poles (50.6957, 16.6373) (50.7747, 16.7479) (50.8601, 17.0671) (50.8601, 17.3453) knots 0 0 0 1 2 2 2
  spline S448 degree 2 poles (53.1798, 15.803) (52.8575, 15.803) (52.2791, 15.9452) (52.0895, 16.04) knots 0 0 0 1 2 2 2
  line L365 (52.0895, 16.04) -> (52.0895, 16.8143)
  line L366 (52.0895, 16.8143) -> (52.1653, 16.8143)
  spline S449 degree 2 poles (52.1653, 16.8143) (52.2317, 16.7637) (52.3992, 16.6436) (52.5477, 16.5773) knots 0 0 0 1 2 2 2
  spline S450 degree 2 poles (52.5477, 16.5773) (52.6773, 16.5172) (52.9965, 16.4319) (53.1862, 16.4319) knots 0 0 0 1 2 2 2
  spline S451 degree 2 poles (53.1862, 16.4319) (53.3789, 16.4319) (53.676, 16.552) (53.676, 16.6816) knots 0 0 0 1 2 2 2
  spline S452 degree 2 poles (53.676, 16.6816) (53.676, 16.7827) (53.5401, 16.8902) (53.3442, 16.9344) knots 0 0 0 1 2 2 2
  spline S453 degree 2 poles (53.3442, 16.9344) (53.2399, 16.9629) (52.9207, 17.0229) (52.7974, 17.0608) knots 0 0 0 1 2 2 2
  spline S454 degree 2 poles (52.7974, 17.0608) (52.4498, 17.1683) (52.1021, 17.5886) (52.1021, 17.9331) knots 0 0 0 1 2 2 2
  spline S455 degree 2 poles (52.1021, 17.9331) (52.1021, 18.1291) (52.2823, 18.4767) (52.4592, 18.6126) knots 0 0 0 1 2 2 2
  spline S456 degree 2 poles (52.4592, 18.6126) (52.6331, 18.7453) (53.1482, 18.9034) (53.4738, 18.9034) knots 0 0 0 1 2 2 2
  spline S457 degree 2 poles (53.4738, 18.9034) (53.7835, 18.9034) (54.3018, 18.7801) (54.4788, 18.6948) knots 0 0 0 1 2 2 2
  line L367 (54.4788, 18.6948) -> (54.4788, 17.9489)
  line L368 (54.4788, 17.9489) -> (54.4061, 17.9489)
  spline S458 degree 2 poles (54.4061, 17.9489) (54.3587, 17.9868) (54.1532, 18.1101) (54.0584, 18.1543) knots 0 0 0 1 2 2 2
  spline S459 degree 2 poles (54.0584, 18.1543) (53.9415, 18.2049) (53.6571, 18.2744) (53.5085, 18.2744) knots 0 0 0 1 2 2 2
  spline S460 degree 2 poles (53.5085, 18.2744) (53.3094, 18.2744) (53.0344, 18.1385) (53.0344, 18.0279) knots 0 0 0 1 2 2 2
  spline S461 degree 2 poles (53.0344, 18.0279) (53.0344, 17.9268) (53.1703, 17.813) (53.3979, 17.7561) knots 0 0 0 1 2 2 2
  spline S462 degree 2 poles (53.3979, 17.7561) (53.5148, 17.7277) (53.8214, 17.674) (53.9636, 17.6265) knots 0 0 0 1 2 2 2
  spline S463 degree 2 poles (53.9636, 17.6265) (54.2797, 17.5254) (54.6084, 17.1304) (54.6084, 16.8017) knots 0 0 0 1 2 2 2
  spline S464 degree 2 poles (54.6084, 16.8017) (54.6084, 16.5962) (54.4156, 16.2201) (54.2354, 16.0937) knots 0 0 0 1 2 2 2
  spline S465 degree 2 poles (54.2354, 16.0937) (54.049, 15.9547) (53.537, 15.803) (53.1798, 15.803) knots 0 0 0 1 2 2 2
  spline S466 degree 2 poles (56.1696, 15.8251) (55.6102, 15.8251) (55.0982, 16.2865) (55.0982, 16.8111) knots 0 0 0 1 2 2 2
  line L369 (55.0982, 16.8111) -> (55.0982, 18.1859)
  line L370 (55.0982, 18.1859) -> (54.7474, 18.1859)
  line L371 (54.7474, 18.1859) -> (54.7474, 18.8244)
  line L372 (54.7474, 18.8244) -> (55.0982, 18.8244)
  line L373 (55.0982, 18.8244) -> (55.0982, 19.665)
  line L374 (55.0982, 19.665) -> (56.0148, 19.665)
  line L375 (56.0148, 19.665) -> (56.0148, 18.8244)
  line L376 (56.0148, 18.8244) -> (56.8997, 18.8244)
  line L377 (56.8997, 18.8244) -> (56.8997, 18.1859)
  line L378 (56.8997, 18.1859) -> (56.0148, 18.1859)
  line L379 (56.0148, 18.1859) -> (56.0148, 17.1398)
  spline S467 degree 2 poles (56.0148, 17.1398) (56.0148, 16.985) (56.0211, 16.7543) (56.059, 16.6626) knots 0 0 0 1 2 2 2
  spline S468 degree 2 poles (56.059, 16.6626) (56.0969, 16.571) (56.2834, 16.4635) (56.4604, 16.4635) knots 0 0 0 1 2 2 2
  spline S469 degree 2 poles (56.4604, 16.4635) (56.5362, 16.4635) (56.7733, 16.5267) (56.8207, 16.552) knots 0 0 0 1 2 2 2
  line L380 (56.8207, 16.552) -> (56.8997, 16.552)
  line L381 (56.8997, 16.552) -> (56.8997, 15.9073)
  spline S470 degree 2 poles (56.8997, 15.9073) (56.7511, 15.8693) (56.4161, 15.8251) (56.1696, 15.8251) knots 0 0 0 1 2 2 2
  spline S471 degree 2 poles (58.8939, 16.1949) (58.7991, 16.1158) (58.6506, 15.9894) (58.5242, 15.9262) knots 0 0 0 1 2 2 2
  spline S472 degree 2 poles (58.5242, 15.9262) (58.4009, 15.8662) (58.167, 15.803) (57.9584, 15.803) knots 0 0 0 1 2 2 2
  spline S473 degree 2 poles (57.9584, 15.803) (57.5665, 15.803) (57.0514, 16.3276) (57.0514, 16.7258) knots 0 0 0 1 2 2 2
  spline S474 degree 2 poles (57.0514, 16.7258) (57.0514, 17.0513) (57.3137, 17.4559) (57.5602, 17.5728) knots 0 0 0 1 2 2 2
  spline S475 degree 2 poles (57.5602, 17.5728) (57.8099, 17.6929) (58.502, 17.7877) (58.9003, 17.813) knots 0 0 0 1 2 2 2
  line L382 (58.9003, 17.813) -> (58.9003, 17.8288)
  spline S476 degree 2 poles (58.9003, 17.8288) (58.9003, 18.0722) (58.54, 18.2586) (58.1797, 18.2586) knots 0 0 0 1 2 2 2
  spline S477 degree 2 poles (58.1797, 18.2586) (58.0185, 18.2586) (57.5823, 18.1417) (57.3769, 18.05) knots 0 0 0 1 2 2 2
  line L383 (57.3769, 18.05) -> (57.2979, 18.05)
  line L384 (57.2979, 18.05) -> (57.2979, 18.7611)
  spline S478 degree 2 poles (57.2979, 18.7611) (57.4338, 18.7991) (58.0406, 18.9065) (58.3503, 18.9065) knots 0 0 0 1 2 2 2
  spline S479 degree 2 poles (58.3503, 18.9065) (59.1088, 18.9065) (59.8041, 18.4009) (59.8041, 17.8825) knots 0 0 0 1 2 2 2
  line L385 (59.8041, 17.8825) -> (59.8041, 15.882)
  line L386 (59.8041, 15.882) -> (58.8939, 15.882)
  line L387 (58.8939, 15.882) -> (58.8939, 16.1949)
  line L388 (58.8939, 16.65) -> (58.8939, 17.2599)
  spline S480 degree 2 poles (58.8939, 17.2599) (58.6601, 17.2378) (58.3725, 17.203) (58.2334, 17.1525) knots 0 0 0 1 2 2 2
  spline S481 degree 2 poles (58.2334, 17.1525) (58.1101, 17.1114) (57.9774, 16.9407) (57.9774, 16.8017) knots 0 0 0 1 2 2 2
  spline S482 degree 2 poles (57.9774, 16.8017) (57.9774, 16.5962) (58.2018, 16.4414) (58.4199, 16.4414) knots 0 0 0 1 2 2 2
  spline S483 degree 2 poles (58.4199, 16.4414) (58.54, 16.4414) (58.7928, 16.552) (58.8939, 16.65) knots 0 0 0 1 2 2 2
  line L389 (64.7186, 19.0393) -> (63.0815, 19.0393)
  line L390 (63.0815, 19.0393) -> (63.0815, 18.3029)
  line L391 (63.0815, 18.3029) -> (64.5891, 18.3029)
  line L392 (64.5891, 18.3029) -> (64.5891, 17.5602)
  line L393 (64.5891, 17.5602) -> (63.0815, 17.5602)
  line L394 (63.0815, 17.5602) -> (63.0815, 15.882)
  line L395 (63.0815, 15.882) -> (62.1081, 15.882)
  line L396 (62.1081, 15.882) -> (62.1081, 19.782)
  line L397 (62.1081, 19.782) -> (64.7186, 19.782)
  line L398 (64.7186, 19.782) -> (64.7186, 19.0393)
  spline S484 degree 2 poles (66.7919, 16.1949) (66.6971, 16.1158) (66.5485, 15.9894) (66.4221, 15.9262) knots 0 0 0 1 2 2 2
  spline S485 degree 2 poles (66.4221, 15.9262) (66.2989, 15.8662) (66.065, 15.803) (65.8564, 15.803) knots 0 0 0 1 2 2 2
  spline S486 degree 2 poles (65.8564, 15.803) (65.4645, 15.803) (64.9494, 16.3276) (64.9494, 16.7258) knots 0 0 0 1 2 2 2
  spline S487 degree 2 poles (64.9494, 16.7258) (64.9494, 17.0513) (65.2117, 17.4559) (65.4582, 17.5728) knots 0 0 0 1 2 2 2
  spline S488 degree 2 poles (65.4582, 17.5728) (65.7079, 17.6929) (66.4, 17.7877) (66.7982, 17.813) knots 0 0 0 1 2 2 2
  line L399 (66.7982, 17.813) -> (66.7982, 17.8288)
  spline S489 degree 2 poles (66.7982, 17.8288) (66.7982, 18.0722) (66.4379, 18.2586) (66.0776, 18.2586) knots 0 0 0 1 2 2 2
  spline S490 degree 2 poles (66.0776, 18.2586) (65.9165, 18.2586) (65.4803, 18.1417) (65.2749, 18.05) knots 0 0 0 1 2 2 2
  line L400 (65.2749, 18.05) -> (65.1959, 18.05)
  line L401 (65.1959, 18.05) -> (65.1959, 18.7611)
  spline S491 degree 2 poles (65.1959, 18.7611) (65.3318, 18.7991) (65.9386, 18.9065) (66.2483, 18.9065) knots 0 0 0 1 2 2 2
  spline S492 degree 2 poles (66.2483, 18.9065) (67.0068, 18.9065) (67.7021, 18.4009) (67.7021, 17.8825) knots 0 0 0 1 2 2 2
  line L402 (67.7021, 17.8825) -> (67.7021, 15.882)
  line L403 (67.7021, 15.882) -> (66.7919, 15.882)
  line L404 (66.7919, 15.882) -> (66.7919, 16.1949)
  line L405 (66.7919, 16.65) -> (66.7919, 17.2599)
  spline S493 degree 2 poles (66.7919, 17.2599) (66.558, 17.2378) (66.2704, 17.203) (66.1314, 17.1525) knots 0 0 0 1 2 2 2
  spline S494 degree 2 poles (66.1314, 17.1525) (66.0081, 17.1114) (65.8754, 16.9407) (65.8754, 16.8017) knots 0 0 0 1 2 2 2
  spline S495 degree 2 poles (65.8754, 16.8017) (65.8754, 16.5962) (66.0998, 16.4414) (66.3178, 16.4414) knots 0 0 0 1 2 2 2
  spline S496 degree 2 poles (66.3178, 16.4414) (66.4379, 16.4414) (66.6908, 16.552) (66.7919, 16.65) knots 0 0 0 1 2 2 2
  line L406 (70.3569, 17.9552) -> (70.281, 17.9552)
  spline S497 degree 2 poles (70.281, 17.9552) (70.2273, 17.9742) (70.0282, 17.9932) (69.9081, 17.9932) knots 0 0 0 1 2 2 2
  spline S498 degree 2 poles (69.9081, 17.9932) (69.7659, 17.9932) (69.4467, 17.9078) (69.2981, 17.8509) knots 0 0 0 1 2 2 2
  line L407 (69.2981, 17.8509) -> (69.2981, 15.882)
  line L408 (69.2981, 15.882) -> (68.3816, 15.882)
  line L409 (68.3816, 15.882) -> (68.3816, 18.8244)
  line L410 (68.3816, 18.8244) -> (69.2981, 18.8244)
  line L411 (69.2981, 18.8244) -> (69.2981, 18.4009)
  spline S499 degree 2 poles (69.2981, 18.4009) (69.3614, 18.4577) (69.5826, 18.6347) (69.6742, 18.6885) knots 0 0 0 1 2 2 2
  spline S500 degree 2 poles (69.6742, 18.6885) (69.7754, 18.7485) (70.0409, 18.8338) (70.1578, 18.8338) knots 0 0 0 1 2 2 2
  spline S501 degree 2 poles (70.1578, 18.8338) (70.202, 18.8338) (70.3126, 18.8275) (70.3569, 18.8244) knots 0 0 0 1 2 2 2
  line L412 (70.3569, 18.8244) -> (70.3569, 17.9552)
  line L413 (71.6242, 15.882) -> (70.7077, 15.882)
  line L414 (70.7077, 15.882) -> (70.7077, 18.8244)
  line L415 (70.7077, 18.8244) -> (71.6242, 18.8244)
  line L416 (71.6242, 18.8244) -> (71.6242, 15.882)
  line L417 (71.6527, 19.2447) -> (70.6824, 19.2447)
  line L418 (70.6824, 19.2447) -> (70.6824, 19.959)
  line L419 (70.6824, 19.959) -> (71.6527, 19.959)
  line L420 (71.6527, 19.959) -> (71.6527, 19.2447)
  spline S502 degree 2 poles (73.9472, 16.1949) (73.8524, 16.1158) (73.7038, 15.9894) (73.5774, 15.9262) knots 0 0 0 1 2 2 2
  spline S503 degree 2 poles (73.5774, 15.9262) (73.4541, 15.8662) (73.2203, 15.803) (73.0117, 15.803) knots 0 0 0 1 2 2 2
  spline S504 degree 2 poles (73.0117, 15.803) (72.6198, 15.803) (72.1046, 16.3276) (72.1046, 16.7258) knots 0 0 0 1 2 2 2
  spline S505 degree 2 poles (72.1046, 16.7258) (72.1046, 17.0513) (72.3669, 17.4559) (72.6135, 17.5728) knots 0 0 0 1 2 2 2
  spline S506 degree 2 poles (72.6135, 17.5728) (72.8631, 17.6929) (73.5553, 17.7877) (73.9535, 17.813) knots 0 0 0 1 2 2 2
  line L421 (73.9535, 17.813) -> (73.9535, 17.8288)
  spline S507 degree 2 poles (73.9535, 17.8288) (73.9535, 18.0722) (73.5932, 18.2586) (73.2329, 18.2586) knots 0 0 0 1 2 2 2
  spline S508 degree 2 poles (73.2329, 18.2586) (73.0717, 18.2586) (72.6356, 18.1417) (72.4302, 18.05) knots 0 0 0 1 2 2 2
  line L422 (72.4302, 18.05) -> (72.3511, 18.05)
  line L423 (72.3511, 18.05) -> (72.3511, 18.7611)
  spline S509 degree 2 poles (72.3511, 18.7611) (72.487, 18.7991) (73.0938, 18.9065) (73.4036, 18.9065) knots 0 0 0 1 2 2 2
  spline S510 degree 2 poles (73.4036, 18.9065) (74.1621, 18.9065) (74.8574, 18.4009) (74.8574, 17.8825) knots 0 0 0 1 2 2 2
  line L424 (74.8574, 17.8825) -> (74.8574, 15.882)
  line L425 (74.8574, 15.882) -> (73.9472, 15.882)
  line L426 (73.9472, 15.882) -> (73.9472, 16.1949)
  line L427 (73.9472, 16.65) -> (73.9472, 17.2599)
  spline S511 degree 2 poles (73.9472, 17.2599) (73.7133, 17.2378) (73.4257, 17.203) (73.2866, 17.1525) knots 0 0 0 1 2 2 2
  spline S512 degree 2 poles (73.2866, 17.1525) (73.1634, 17.1114) (73.0306, 16.9407) (73.0306, 16.8017) knots 0 0 0 1 2 2 2
  spline S513 degree 2 poles (73.0306, 16.8017) (73.0306, 16.5962) (73.255, 16.4414) (73.4731, 16.4414) knots 0 0 0 1 2 2 2
  spline S514 degree 2 poles (73.4731, 16.4414) (73.5932, 16.4414) (73.846, 16.552) (73.9472, 16.65) knots 0 0 0 1 2 2 2
  spline S515 degree 2 poles (11.6219, 12.1058) (11.6219, 11.834) (11.4481, 11.341) (11.2869, 11.1766) knots 0 0 0 1 2 2 2
  spline S516 degree 2 poles (11.2869, 11.1766) (11.1889, 11.0723) (10.9487, 10.9017) (10.8065, 10.8416) knots 0 0 0 1 2 2 2
  spline S517 degree 2 poles (10.8065, 10.8416) (10.6611, 10.7816) (10.3229, 10.712) (10.1143, 10.712) knots 0 0 0 1 2 2 2
  line L428 (10.1143, 10.712) -> (9.6024, 10.712)
  line L429 (9.6024, 10.712) -> (9.6024, 9.4352)
  line L430 (9.6024, 9.4352) -> (8.6226, 9.4352)
  line L431 (8.6226, 9.4352) -> (8.6226, 13.3352)
  line L432 (8.6226, 13.3352) -> (10.1365, 13.3352)
  spline S518 degree 2 poles (10.1365, 13.3352) (10.4715, 13.3352) (10.9613, 13.212) (11.1605, 13.0792) knots 0 0 0 1 2 2 2
  spline S519 degree 2 poles (11.1605, 13.0792) (11.3817, 12.9307) (11.6219, 12.444) (11.6219, 12.1058) knots 0 0 0 1 2 2 2
  spline S520 degree 2 poles (10.6169, 12.0805) (10.6169, 12.248) (10.4588, 12.4851) (10.3514, 12.5293) knots 0 0 0 1 2 2 2
  spline S521 degree 2 poles (10.3514, 12.5293) (10.2123, 12.5894) (9.9595, 12.6083) (9.7414, 12.6083) knots 0 0 0 1 2 2 2
  line L433 (9.7414, 12.6083) -> (9.6024, 12.6083)
  line L434 (9.6024, 12.6083) -> (9.6024, 11.4389)
  line L435 (9.6024, 11.4389) -> (9.6719, 11.4389)
  spline S522 degree 2 poles (9.6719, 11.4389) (9.8078, 11.4389) (10.0543, 11.4453) (10.1459, 11.4611) knots 0 0 0 1 2 2 2
  spline S523 degree 2 poles (10.1459, 11.4611) (10.225, 11.4737) (10.3988, 11.5496) (10.4462, 11.597) knots 0 0 0 1 2 2 2
  spline S524 degree 2 poles (10.4462, 11.597) (10.5473, 11.6918) (10.6169, 11.9035) (10.6169, 12.0805) knots 0 0 0 1 2 2 2
  line L436 (14.0681, 11.5085) -> (13.9922, 11.5085)
  spline S525 degree 2 poles (13.9922, 11.5085) (13.9385, 11.5274) (13.7394, 11.5464) (13.6193, 11.5464) knots 0 0 0 1 2 2 2
  spline S526 degree 2 poles (13.6193, 11.5464) (13.4771, 11.5464) (13.1579, 11.4611) (13.0093, 11.4042) knots 0 0 0 1 2 2 2
  line L437 (13.0093, 11.4042) -> (13.0093, 9.4352)
  line L438 (13.0093, 9.4352) -> (12.0928, 9.4352)
  line L439 (12.0928, 9.4352) -> (12.0928, 12.3776)
  line L440 (12.0928, 12.3776) -> (13.0093, 12.3776)
  line L441 (13.0093, 12.3776) -> (13.0093, 11.9541)
  spline S527 degree 2 poles (13.0093, 11.9541) (13.0725, 12.011) (13.2938, 12.188) (13.3854, 12.2417) knots 0 0 0 1 2 2 2
  spline S528 degree 2 poles (13.3854, 12.2417) (13.4865, 12.3018) (13.752, 12.3871) (13.869, 12.3871) knots 0 0 0 1 2 2 2
  spline S529 degree 2 poles (13.869, 12.3871) (13.9132, 12.3871) (14.0238, 12.3808) (14.0681, 12.3776) knots 0 0 0 1 2 2 2
  line L442 (14.0681, 12.3776) -> (14.0681, 11.5085)
  spline S530 degree 2 poles (17.2412, 10.9048) (17.2412, 10.1779) (16.4479, 9.3436) (15.7241, 9.3436) knots 0 0 0 1 2 2 2
  spline S531 degree 2 poles (15.7241, 9.3436) (15.0036, 9.3436) (14.204, 10.1779) (14.204, 10.9048) knots 0 0 0 1 2 2 2
  spline S532 degree 2 poles (14.204, 10.9048) (14.204, 11.6381) (15.0036, 12.4693) (15.7241, 12.4693) knots 0 0 0 1 2 2 2
  spline S533 degree 2 poles (15.7241, 12.4693) (16.4447, 12.4693) (17.2412, 11.6349) (17.2412, 10.9048) knots 0 0 0 1 2 2 2
  spline S534 degree 2 poles (16.3025, 10.8985) (16.3025, 11.1608) (16.2172, 11.5116) (16.1413, 11.6159) knots 0 0 0 1 2 2 2
  spline S535 degree 2 poles (16.1413, 11.6159) (16.0592, 11.7265) (15.8537, 11.8119) (15.7241, 11.8119) knots 0 0 0 1 2 2 2
  spline S536 degree 2 poles (15.7241, 11.8119) (15.5977, 11.8119) (15.3986, 11.736) (15.3165, 11.6286) knots 0 0 0 1 2 2 2
  spline S537 degree 2 poles (15.3165, 11.6286) (15.2374, 11.5274) (15.1426, 11.1703) (15.1426, 10.8985) knots 0 0 0 1 2 2 2
  spline S538 degree 2 poles (15.1426, 10.8985) (15.1426, 10.6299) (15.2311, 10.298) (15.3038, 10.1969) knots 0 0 0 1 2 2 2
  spline S539 degree 2 poles (15.3038, 10.1969) (15.3765, 10.0958) (15.5977, 10.0009) (15.7305, 10.0009) knots 0 0 0 1 2 2 2
  spline S540 degree 2 poles (15.7305, 10.0009) (15.8411, 10.0009) (16.0686, 10.0958) (16.1382, 10.1906) knots 0 0 0 1 2 2 2
  spline S541 degree 2 poles (16.1382, 10.1906) (16.2172, 10.3012) (16.3025, 10.6204) (16.3025, 10.8985) knots 0 0 0 1 2 2 2
  line L443 (19.6083, 12.8169) -> (19.5388, 12.8169)
  spline S542 degree 2 poles (19.5388, 12.8169) (19.4851, 12.8327) (19.2607, 12.8833) (19.1627, 12.8833) knots 0 0 0 1 2 2 2
  spline S543 degree 2 poles (19.1627, 12.8833) (18.8846, 12.8833) (18.6823, 12.681) (18.6823, 12.3997) knots 0 0 0 1 2 2 2
  line L444 (18.6823, 12.3997) -> (18.6823, 12.3776)
  line L445 (18.6823, 12.3776) -> (19.4124, 12.3776)
  line L446 (19.4124, 12.3776) -> (19.4124, 11.7392)
  line L447 (19.4124, 11.7392) -> (18.7139, 11.7392)
  line L448 (18.7139, 11.7392) -> (18.7139, 9.4352)
  line L449 (18.7139, 9.4352) -> (17.7974, 9.4352)
  line L450 (17.7974, 9.4352) -> (17.7974, 11.7392)
  line L451 (17.7974, 11.7392) -> (17.4308, 11.7392)
  line L452 (17.4308, 11.7392) -> (17.4308, 12.3776)
  line L453 (17.4308, 12.3776) -> (17.7974, 12.3776)
  line L454 (17.7974, 12.3776) -> (17.7974, 12.4598)
  spline S544 degree 2 poles (17.7974, 12.4598) (17.7974, 12.9971) (18.3631, 13.5343) (18.9383, 13.5343) knots 0 0 0 1 2 2 2
  spline S545 degree 2 poles (18.9383, 13.5343) (19.1374, 13.5343) (19.4819, 13.5059) (19.6083, 13.4806) knots 0 0 0 1 2 2 2
  line L455 (19.6083, 13.4806) -> (19.6083, 12.8169)
  line L456 (20.7271, 9.4352) -> (19.8011, 9.4352)
  line L457 (19.8011, 9.4352) -> (19.8011, 10.4655)
  line L458 (19.8011, 10.4655) -> (20.7271, 10.4655)
  line L459 (20.7271, 10.4655) -> (20.7271, 9.4352)
  spline S546 degree 2 poles (26.5582, 11.3821) (26.5582, 10.8353) (26.081, 9.9757) (25.7175, 9.7449) knots 0 0 0 1 2 2 2
  spline S547 degree 2 poles (25.7175, 9.7449) (25.4141, 9.549) (24.6998, 9.4352) (24.2985, 9.4352) knots 0 0 0 1 2 2 2
  line L460 (24.2985, 9.4352) -> (23.0785, 9.4352)
  line L461 (23.0785, 9.4352) -> (23.0785, 13.3352)
  line L462 (23.0785, 13.3352) -> (24.2858, 13.3352)
  spline S548 degree 2 poles (24.2858, 13.3352) (24.6967, 13.3352) (25.4141, 13.2309) (25.7301, 13.0287) knots 0 0 0 1 2 2 2
  spline S549 degree 2 poles (25.7301, 13.0287) (26.1126, 12.7821) (26.5582, 11.9478) (26.5582, 11.3821) knots 0 0 0 1 2 2 2
  spline S550 degree 2 poles (25.5532, 11.3884) (25.5532, 11.774) (25.2877, 12.3239) (25.0159, 12.4787) knots 0 0 0 1 2 2 2
  spline S551 degree 2 poles (25.0159, 12.4787) (24.8168, 12.5862) (24.3806, 12.6083) (24.0772, 12.6083) knots 0 0 0 1 2 2 2
  line L463 (24.0772, 12.6083) -> (24.0583, 12.6083)
  line L464 (24.0583, 12.6083) -> (24.0583, 10.1653)
  line L465 (24.0583, 10.1653) -> (24.0772, 10.1653)
  spline S552 degree 2 poles (24.0772, 10.1653) (24.4059, 10.1653) (24.8579, 10.1874) (25.0633, 10.317) knots 0 0 0 1 2 2 2
  spline S553 degree 2 poles (25.0633, 10.317) (25.3035, 10.4687) (25.5532, 11.0028) (25.5532, 11.3884) knots 0 0 0 1 2 2 2
  line L466 (29.0613, 11.5085) -> (28.9854, 11.5085)
  spline S554 degree 2 poles (28.9854, 11.5085) (28.9317, 11.5274) (28.7326, 11.5464) (28.6125, 11.5464) knots 0 0 0 1 2 2 2
  spline S555 degree 2 poles (28.6125, 11.5464) (28.4703, 11.5464) (28.1511, 11.4611) (28.0025, 11.4042) knots 0 0 0 1 2 2 2
  line L467 (28.0025, 11.4042) -> (28.0025, 9.4352)
  line L468 (28.0025, 9.4352) -> (27.086, 9.4352)
  line L469 (27.086, 9.4352) -> (27.086, 12.3776)
  line L470 (27.086, 12.3776) -> (28.0025, 12.3776)
  line L471 (28.0025, 12.3776) -> (28.0025, 11.9541)
  spline S556 degree 2 poles (28.0025, 11.9541) (28.0657, 12.011) (28.287, 12.188) (28.3786, 12.2417) knots 0 0 0 1 2 2 2
  spline S557 degree 2 poles (28.3786, 12.2417) (28.4797, 12.3018) (28.7452, 12.3871) (28.8622, 12.3871) knots 0 0 0 1 2 2 2
  spline S558 degree 2 poles (28.8622, 12.3871) (28.9064, 12.3871) (29.017, 12.3808) (29.0613, 12.3776) knots 0 0 0 1 2 2 2
  line L472 (29.0613, 12.3776) -> (29.0613, 11.5085)
  line L473 (30.3602, 9.4352) -> (29.4342, 9.4352)
  line L474 (29.4342, 9.4352) -> (29.4342, 10.4655)
  line L475 (29.4342, 10.4655) -> (30.3602, 10.4655)
  line L476 (30.3602, 10.4655) -> (30.3602, 9.4352)
  line L477 (35.3221, 12.5925) -> (33.685, 12.5925)
  line L478 (33.685, 12.5925) -> (33.685, 11.8561)
  line L479 (33.685, 11.8561) -> (35.1925, 11.8561)
  line L480 (35.1925, 11.8561) -> (35.1925, 11.1134)
  line L481 (35.1925, 11.1134) -> (33.685, 11.1134)
  line L482 (33.685, 11.1134) -> (33.685, 9.4352)
  line L483 (33.685, 9.4352) -> (32.7116, 9.4352)
  line L484 (32.7116, 9.4352) -> (32.7116, 13.3352)
  line L485 (32.7116, 13.3352) -> (35.3221, 13.3352)
  line L486 (35.3221, 13.3352) -> (35.3221, 12.5925)
  line L487 (36.6906, 9.4352) -> (35.7741, 9.4352)
  line L488 (35.7741, 9.4352) -> (35.7741, 13.509)
  line L489 (35.7741, 13.509) -> (36.6906, 13.509)
  line L490 (36.6906, 13.509) -> (36.6906, 9.4352)
  spline S559 degree 2 poles (39.0135, 9.7481) (38.9187, 9.6691) (38.7702, 9.5427) (38.6438, 9.4795) knots 0 0 0 1 2 2 2
  spline S560 degree 2 poles (38.6438, 9.4795) (38.5205, 9.4194) (38.2866, 9.3562) (38.078, 9.3562) knots 0 0 0 1 2 2 2
  spline S561 degree 2 poles (38.078, 9.3562) (37.6861, 9.3562) (37.171, 9.8808) (37.171, 10.2791) knots 0 0 0 1 2 2 2
  spline S562 degree 2 poles (37.171, 10.2791) (37.171, 10.6046) (37.4333, 11.0091) (37.6798, 11.1261) knots 0 0 0 1 2 2 2
  spline S563 degree 2 poles (37.6798, 11.1261) (37.9295, 11.2462) (38.6216, 11.341) (39.0199, 11.3663) knots 0 0 0 1 2 2 2
  line L491 (39.0199, 11.3663) -> (39.0199, 11.3821)
  spline S564 degree 2 poles (39.0199, 11.3821) (39.0199, 11.6254) (38.6596, 11.8119) (38.2993, 11.8119) knots 0 0 0 1 2 2 2
  spline S565 degree 2 poles (38.2993, 11.8119) (38.1381, 11.8119) (37.7019, 11.6949) (37.4965, 11.6033) knots 0 0 0 1 2 2 2
  line L492 (37.4965, 11.6033) -> (37.4175, 11.6033)
  line L493 (37.4175, 11.6033) -> (37.4175, 12.3144)
  spline S566 degree 2 poles (37.4175, 12.3144) (37.5534, 12.3523) (38.1602, 12.4598) (38.4699, 12.4598) knots 0 0 0 1 2 2 2
  spline S567 degree 2 poles (38.4699, 12.4598) (39.2284, 12.4598) (39.9237, 11.9541) (39.9237, 11.4358) knots 0 0 0 1 2 2 2
  line L494 (39.9237, 11.4358) -> (39.9237, 9.4352)
  line L495 (39.9237, 9.4352) -> (39.0135, 9.4352)
  line L496 (39.0135, 9.4352) -> (39.0135, 9.7481)
  line L497 (39.456, 13.8251) -> (38.669, 12.7948)
  line L498 (38.669, 12.7948) -> (38.0464, 12.7948)
  line L499 (38.0464, 12.7948) -> (38.59, 13.8251)
  line L500 (38.59, 13.8251) -> (39.456, 13.8251)
  line L501 (39.0135, 10.2032) -> (39.0135, 10.8132)
  spline S568 degree 2 poles (39.0135, 10.8132) (38.7797, 10.7911) (38.4921, 10.7563) (38.353, 10.7057) knots 0 0 0 1 2 2 2
  spline S569 degree 2 poles (38.353, 10.7057) (38.2297, 10.6646) (38.097, 10.494) (38.097, 10.3549) knots 0 0 0 1 2 2 2
  spline S570 degree 2 poles (38.097, 10.3549) (38.097, 10.1495) (38.3214, 9.9946) (38.5395, 9.9946) knots 0 0 0 1 2 2 2
  spline S571 degree 2 poles (38.5395, 9.9946) (38.6596, 9.9946) (38.9124, 10.1052) (39.0135, 10.2032) knots 0 0 0 1 2 2 2
  line L502 (43.356, 12.3776) -> (42.3004, 9.4352)
  line L503 (42.3004, 9.4352) -> (41.2985, 9.4352)
  line L504 (41.2985, 9.4352) -> (40.2524, 12.3776)
  line L505 (40.2524, 12.3776) -> (41.2164, 12.3776)
  line L506 (41.2164, 12.3776) -> (41.8169, 10.4339)
  line L507 (41.8169, 10.4339) -> (42.411, 12.3776)
  line L508 (42.411, 12.3776) -> (43.356, 12.3776)
  line L509 (44.6233, 9.4352) -> (43.7068, 9.4352)
  line L510 (43.7068, 9.4352) -> (43.7068, 12.3776)
  line L511 (43.7068, 12.3776) -> (44.6233, 12.3776)
  line L512 (44.6233, 12.3776) -> (44.6233, 9.4352)
  line L513 (44.6518, 12.7979) -> (43.6815, 12.7979)
  line L514 (43.6815, 12.7979) -> (43.6815, 13.5122)
  line L515 (43.6815, 13.5122) -> (44.6518, 13.5122)
  line L516 (44.6518, 13.5122) -> (44.6518, 12.7979)